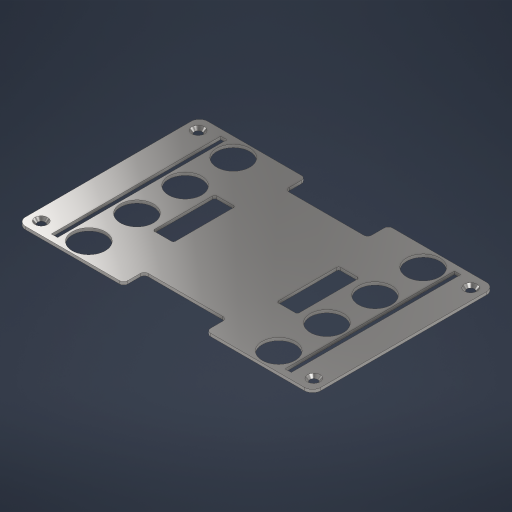
# Autodesk Inventor part: spacer
Saved by Autodesk Inventor 2024 (Build 280153000, 153)
## iProperties
Created: 2021-07-16
Part Number: spacer
Material: Stainless Steel
Document SubType Name: Modeling
Designer: Caleb
Density: 8 g/cm^3
Appearance: Semi-Polished
Author: Caleb
Autodesk Inventor part; units mm, degrees
ref_plane "YZ Plane" through (0, 0, 0) normal (1, 0, 0) x (0, 1, 0)
ref_plane "XZ Plane" through (0, 0, 0) normal (0, 1, 0) x (-1, 0, 0)
ref_plane "XY Plane" through (0, 0, 0) normal (0, 0, 1) x (1, 0, 0)
sketch "Sketch1" plane through (0, 0, 0) normal (0, 1, 0) x (-1, 0, 0)
  line L0 (-35.75, 22.05) -> (35.75, 22.05)
  line L1 (35.75, 22.05) -> (35.75, -22.05)
  line L2 (35.75, -22.05) -> (-35.75, -22.05)
  line L3 (-35.75, -22.05) -> (-35.75, 22.05)
  line L4 (-35.75, 22.05) -> (35.75, -22.05) construction
  line L5 (35.75, 22.05) -> (-35.75, -22.05) construction
  point P0 (0, 0)
  dimension "d0" = 44.1
  dimension "d1" = 71.5
  constraints: 12 end point, 8 point on line, 2 midpoint, 2 parallel, 1 horizontal, 1 perpendicular
  measures "d0" distance of L5.start L4.end
  measures "d1" distance of L4.end L5.end
extrude "Extrusion1" add sketch "Sketch1" along normal blind 0.7
sketch "Sketch2" plane through (0, 0.7, 0) normal (0, 1, 0) x (1, 0, 0)
  point P0 (0, 0)
  point P1 (-33, 19)
  point P2 (33, 19)
  point P3 (-33, -19)
  point P4 (33, -19)
  dimension "d77" = 38
  dimension "d78" = 19
  dimension "d79" = 33
  dimension "d115" = 33
  constraints: 2 horizontal alignment, 2 vertical alignment
  measures "d77" distance of point (-33, -19) point (-33, 19)
  measures "d78" vertical distance of point (-33, 19) point (0, 0)
  measures "d79" horizontal distance of point (-33, 19) point (0, 0)
  measures "d115" horizontal distance of point (0, 0) point (33, 19)
hole "Hole1" at (-33, 0.7, -19) at (33, 0.7, -19) at (-33, 0.7, 19) at (33, 0.7, 19) direction (0, -1, 0) diameter 1.778 end through all countersink diameter 3.023 countersink angle 82 clearance for "Flat Head Machine Screw (82)" size "#0" standard "Ansi Unified Screw Threads"
sketch "Sketch3" plane through (0, 0.7, 0) normal (0, 1, 0) x (1, 0, 0)
  line L0 (-13, -7.5) -> (-17, -7.5)
  line L1 (-17.5, -7) -> (-17.5, 7)
  line L2 (-17, 7.5) -> (-13, 7.5)
  line L3 (-12.5, -7.5) -> (-17.5, 7.5) construction
  line L4 (-17.5, -7.5) -> (-12.5, 7.5) construction
  line L5 (17, -7.5) -> (13, -7.5)
  line L6 (13, 7.5) -> (17, 7.5)
  line L7 (17.5, 7) -> (17.5, -7)
  line L8 (17.5, -7.5) -> (12.5, 7.5) construction
  line L9 (12.5, -7.5) -> (17.5, 7.5) construction
  arc A0 (-17.5, -7) -> (-17, -7.5) centre (-17, -7) ccw
  arc A1 (-17, 7.5) -> (-17.5, 7) centre (-17, 7) ccw
  arc A2 (17, -7.5) -> (17.5, -7) centre (17, -7) ccw
  arc A3 (17.5, 7) -> (17, 7.5) centre (17, 7) ccw
  line L10 (-12.5, 7) -> (-12.5, -7)
  arc A4 (-13, -7.5) -> (-12.5, -7) centre (-13, -7) ccw
  arc A5 (-12.5, 7) -> (-13, 7.5) centre (-13, 7) ccw
  line L11 (12.5, 7) -> (12.5, -7)
  arc A6 (12.5, -7) -> (13, -7.5) centre (13, -7) ccw
  arc A7 (13, 7.5) -> (12.5, 7) centre (13, 7) ccw
  point P0 (0, 0)
  point P1 (-15, 0)
  point P2 (15, 0)
  point P3 (-15, 0)
  point P4 (15, 0)
  point P5 (-15, 0)
  dimension "d18" = 15
  dimension "d21" = 5
  dimension "d72" = 30
  dimension "d73" = 15
  dimension "d85" = 0.5
  dimension "d88" = 0.5
  dimension "d89" = 0.5
  dimension "d90" = 0.5
  dimension "d91" = 5
  dimension "d92" = 15
  constraints: 24 end point, 20 point on line, 16 point on circle, 16 tangent, 8 centre point, 7 midpoint, 3 parallel, 2 equal radius, 2 horizontal, 2 horizontal alignment, 2 vertical, 1 coincident, 1 collinear, 1 perpendicular
  measures "d18" distance of L4.start L3.end
  measures "d21" distance of L3.start L4.start
  measures "d72" distance of point (15, 0) point (-15, 0)
  measures "d73" distance of point (-15, 0) point (0, 0)
  measures "d85" radius of A0
  measures "d88" radius of A1
  measures "d89" radius of A4
  measures "d90" radius of A6
  measures "d91" distance between parallel lines of L7 L11
  measures "d92" distance between parallel lines of L6 L5
extrude "Extrusion2" cut sketch "Sketch3" against normal through all
sketch "Sketch8" plane through (0, 0.7, 0) normal (0, 1, 0) x (1, 0, 0)
  line L0 (0, -25.8162) -> (0, 35.4603)
  line L1 (35.75, -22.05) -> (35.75, 22.05) projected
  point P0 (0, 0)
  point P1 (23, -5.8333)
  point P2 (23, 5.8333)
  point P3 (23, -17.5)
  point P4 (23, 17.5)
  point P5 (-23, -5.8333)
  point P6 (-23, 5.8333)
  point P7 (-23, -17.5)
  point P8 (-23, 17.5)
  dimension "d101" = 5.8333
  dimension "d102" = 5.8333
  dimension "d103" = 11.6667
  dimension "d104" = 11.6667
  dimension "d113" = 23
  constraints: 4 symmetric about line, 3 vertical alignment, 2 end point, 1 point on line, 1 vertical
  measures "d101" vertical distance of point (0, 0) point (23, -5.833)
  measures "d102" vertical distance of point (0, 0) point (23, 5.833)
  measures "d103" distance of point (23, -5.833) point (23, -17.5)
  measures "d104" distance of point (23, 5.833) point (23, 17.5)
  measures "d113" horizontal distance of point (23, -17.5) point (0, 0)
hole "Hole4" at (23, 0.7, 5.8333) at (23, 0.7, -5.8333) at (23, 0.7, 17.5) at (23, 0.7, -17.5) at (-23, 0.7, 17.5) at (-23, 0.7, 5.8333) at (-23, 0.7, -5.8333) at (-23, 0.7, -17.5) direction (0, -1, 0) diameter 8 end through all
fillet "Fillet3" radius 2 4 edges at (35.75, 0.35, 22.05) (35.75, 0.35, -22.05) (-35.75, 0.35, -22.05) (-35.75, 0.35, 22.05)
sketch "Sketch9" plane through (0, 0.7, 0) normal (0, 1, 0) x (1, 0, 0)
  line L0 (10, -21.05) -> (10, -18.05)
  line L1 (9, -17.05) -> (-9, -17.05)
  line L2 (-10, -18.05) -> (-10, -21.05)
  arc A0 (-9, -17.05) -> (-10, -18.05) centre (-9, -18.05) ccw
  arc A1 (10, -18.05) -> (9, -17.05) centre (9, -18.05) ccw
  line L3 (14.7633, -22.05) -> (11, -22.05)
  arc A2 (10, -21.05) -> (11, -22.05) centre (11, -21.05) ccw
  line L4 (-11, -22.05) -> (-14.1799, -22.05)
  line L5 (-33.75, -22.05) -> (33.75, -22.05) projected
  arc A3 (-11, -22.05) -> (-10, -21.05) centre (-11, -21.05) ccw
  line L6 (-33.75, -22.05) -> (33.75, -22.05) projected
  line L7 (-35.75, 20.05) -> (-35.75, -20.05) projected
  line L8 (-30.6342, 0) -> (24.5057, 0)
  line L9 (10, 21.05) -> (10, 18.05)
  line L10 (9, 17.05) -> (-9, 17.05)
  line L11 (-10, 18.05) -> (-10, 21.05)
  arc A4 (-10, 18.05) -> (-9, 17.05) centre (-9, 18.05) ccw
  arc A5 (9, 17.05) -> (10, 18.05) centre (9, 18.05) ccw
  line L12 (14.7633, 22.05) -> (11, 22.05)
  arc A6 (11, 22.05) -> (10, 21.05) centre (11, 21.05) ccw
  line L13 (-11, 22.05) -> (-14.1799, 22.05)
  line L14 (-33.75, 22.05) -> (33.75, 22.05)
  arc A7 (-10, 21.05) -> (-11, 22.05) centre (-11, 21.05) ccw
  line L15 (-33.75, 22.05) -> (33.75, 22.05)
  point P0 (0, 0)
  point P1 (-10, -22.05)
  point P2 (10, -17.05)
  point P3 (-10, -17.05)
  point P4 (-10, 22.05)
  point P5 (10, 17.05)
  point P6 (-10, 17.05)
  dimension "d116" = 5
  dimension "d117" = 20
  dimension "d118" = 10
  dimension "d119" = 1
  dimension "d120" = 1
  dimension "d121" = 1
  constraints: 26 end point, 19 symmetric about line, 16 point on circle, 16 point on line, 8 centre point, 8 tangent, 3 parallel, 2 collinear, 1 equal radius, 1 horizontal, 4 other
  measures "d116" distance of point (-10, -17.05) point (-10, -22.05)
  measures "d117" distance of point (10, -17.05) point (-10, -17.05)
  measures "d118" distance from line of L2 point (0, 0)
  measures "d119" radius of A0
  measures "d120" radius of A2
  measures "d121" radius of A3
extrude "Extrusion6" cut sketch "Sketch9" against normal through all
sketch "Sketch10" plane through (0, 0.7, 0) normal (0, 1, 0) x (1, 0, 0)
  line L0 (-27.55, -20.5) -> (-29.05, -20.5)
  line L1 (-29.05, -20.5) -> (-29.05, 20.5)
  line L2 (-29.05, 20.5) -> (-27.55, 20.5)
  line L3 (-27.55, 20.5) -> (-27.55, -20.5)
  line L4 (-27.55, -20.5) -> (-29.05, 20.5) construction
  line L5 (-29.05, -20.5) -> (-27.55, 20.5) construction
  line L6 (0, 13.6561) -> (0, -11.4856)
  line L7 (27.55, -20.5) -> (29.05, -20.5)
  line L8 (29.05, -20.5) -> (29.05, 20.5)
  line L9 (29.05, 20.5) -> (27.55, 20.5)
  line L10 (27.55, 20.5) -> (27.55, -20.5)
  line L11 (27.55, -20.5) -> (29.05, 20.5) construction
  line L12 (29.05, -20.5) -> (27.55, 20.5) construction
  point P0 (0, 0)
  point P1 (-28.3, 0)
  point P2 (-27.55, 0)
  point P3 (28.3, 0)
  point P4 (27.55, 0)
  dimension "d124" = 1.5
  dimension "d125" = 41
  dimension "d126" = 27.55
  constraints: 26 end point, 6 symmetric about line, 3 midpoint, 2 parallel, 1 horizontal, 1 horizontal alignment, 1 perpendicular, 1 point on line, 1 vertical
  measures "d124" distance of L1.end L2.end
  measures "d125" distance of L0.end L1.end
  measures "d126" distance of point (0, 0) point (-27.55, 0)
extrude "Extrusion7" cut sketch "Sketch10" against normal through all
equation "\"d78\" = 0.5 * d77"
equation "\"d115\" = d79"
equation "\"d73\" = 0.5 * d72"
equation "\"d88\" = d85"
equation "\"d89\" = d85"
equation "\"d90\" = d85"
equation "\"d91\" = d21"
equation "\"d92\" = d18"
equation "\"d102\" = d101"
equation "\"d104\" = d103"
equation "\"d118\" = 0.5 * d117"
body "Solid1"
